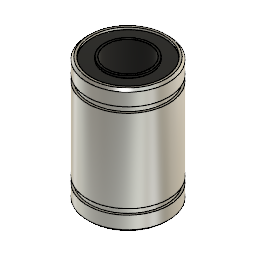
LM10UU_F01 (Autodesk Fusion 360 design; units mm, degrees)
Autodesk Fusion 360 part; units mm, degrees
sketch "スケッチ1" plane through (0, 0, 0) normal (0, 1, 0) x (1, 0, 0)
  line L0 (0, 0) -> (0, -14.5)
  line L1 (0, -14.5) -> (9.5, -14.5)
  line L2 (9.5, -14.5) -> (9.5, -11)
  line L3 (9.5, -11) -> (9, -11)
  line L4 (9, -11) -> (9, -9.7)
  line L5 (9, -9.7) -> (9.5, -9.7)
  line L6 (9.5, -9.7) -> (9.5, 9.7)
  line L7 (9.5, 9.7) -> (9, 9.7)
  line L8 (9, 9.7) -> (9, 11)
  line L9 (9, 11) -> (9.5, 11)
  line L10 (9.5, 11) -> (9.5, 14.5)
  line L11 (9.5, 14.5) -> (0, 14.5)
  line L12 (0, 14.5) -> (0, 0)
  line L13 (8.5, -14.5) -> (8.5, 14.5)
  line L14 (5.5, -14.5) -> (5.5, -14)
  line L15 (5.5, -14) -> (8.5, -14)
  line L16 (5, -14.5) -> (5, 14.5)
  line L17 (5.5, 14.5) -> (5.5, 14)
  line L18 (5.5, 14) -> (8.5, 14)
  dimension "d1" = 9.5
  dimension "d2" = 14.5
  dimension "d3" = 14.5
  dimension "d4" = 9
  dimension "d5" = 3.5
  dimension "d6" = 1.3
  dimension "d7" = 3.5
  dimension "d8" = 1.3
  dimension "d9" = 8.5
  dimension "d10" = 5
  dimension "d11" = 0.5
  dimension "d12" = 0.5
  dimension "d13" = 0.5
  measures "d1" distance of L0 L2
  measures "d2" distance of L0.start L1
  measures "d3" distance of L0.start L11
  measures "d4" distance of L0 L4
  measures "d5" distance of L1 L3
  measures "d9" distance of L0 L13
  measures "d10" distance of L0 L16
  measures "d11" distance of L14 L16
revolve "回転1" add sketch "スケッチ1" angle 360 about axis through (0, 0, 0) along (0, 0, 1) contours L1 L11 L13 L14 L15 L16 L17 L18 makes body 1
revolve "回転2" add sketch "スケッチ1" angle 360 about axis through (0, 0, 1.75) along (0, 0, 1) separate body contours L1 L2 L3 L4 L5 L6 L7 L8 L9 L10 L11 L13 makes body 2
chamfer "面取り1" distance 0.5 angle 45 2 edges at (-8.8571, -3.4353, 14.5) (-8.8571, -3.4353, -14.5) on bodies 2
equation "d3 = d2"
equation "d7 = d5"
equation "d8 = d6"
equation "d13 = d12"
